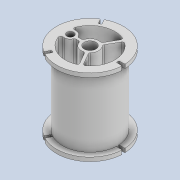
# Autodesk Inventor part: roller_3
Saved by Autodesk Inventor 2020 (Build 240168000, 168)
## iProperties
Created: 2021-09-21
Part Number: roller_3
Material: Generic
Document SubType Name: Modeling
Designer: Shuang Peng
Density: 1 g/cm^3
Appearance: Default
Author: Shuang Peng
Autodesk Inventor part; units mm, degrees
ref_plane "YZ Plane" through (0, 0, 0) normal (1, 0, 0) x (0, 1, 0)
ref_plane "XZ Plane" through (0, 0, 0) normal (0, 1, 0) x (-1, 0, 0)
ref_plane "XY Plane" through (0, 0, 0) normal (0, 0, 1) x (1, 0, 0)
sketch "Sketch1" plane through (0, 0, 0) normal (0, 1, 0) x (-1, 0, 0)
  circle A0 centre (0, 0) radius 7
  circle A1 centre (0, 0) radius 1.5
  circle A2 centre (0, 0) radius 2.2
  circle A3 centre (0, 0) radius 6.3
  line L0 (0, 0) -> (7, 0)
  line L1 (7, 0) -> (0, 0) construction
  line L2 (7, 0.35) -> (0, 0.35)
  line L3 (0, -0.35) -> (7, -0.35)
  arc A4 (7, -0.35) -> (7, 0.35) centre (7, 0) ccw
  arc A5 (0, 0.35) -> (0, -0.35) centre (0, 0) ccw
  line L4 (0.3031, 0.175) -> (-3.1969, 6.2372)
  line L5 (-3.8031, 5.8872) -> (-0.3031, -0.175)
  line L6 (-0.3031, 0.175) -> (-3.8031, -5.8872)
  line L7 (-3.1969, -6.2372) -> (0.3031, -0.175)
  line L8 (0, 0) -> (5, 0)
  circle A6 centre (5, 0) radius 1.5
  line L9 (5, 1.5) -> (6.1188, 1.5)
  line L10 (5, -1.5) -> (6.1188, -1.5)
  line L11 (5, 0) -> (5, -1.5)
  line L12 (5, 0) -> (5, 1.5)
  point P0 (3.5, 0)
  point P1 (-0.7829, 2.056)
  point P2 (-2.842, 5.6225)
  point P3 (3.5414, 0.35)
  point P4 (2.172, 0.35)
  point P5 (-1.3891, 1.706)
  point P6 (-1.3891, -1.706)
  point P7 (-3.4482, -5.2725)
  point P8 (-3.4482, 5.2725)
  point P9 (-2.842, -5.6225)
  point P10 (-0.7829, -2.056)
  point P11 (2.172, -0.35)
  point P12 (3.5414, -0.35)
  dimension "d0" = 14
  dimension "d1" = 3
  dimension "d2" = 0.7
  dimension "d3" = 0.7
  dimension "d4" = 3.5
  dimension "d5" = 0.7
  dimension "d8" = 360
  dimension "d10" = 5
  dimension "d11" = 3
  constraints: 28 end point, 8 point on circle, 6 centre point, 5 coincident, 4 tangent, 2 horizontal, 2 midpoint, 2 parallel, 1 collinear, 1 horizontal alignment, 1 perpendicular, 1 point on line, 1 vertical, 21 other
  measures "d1" diameter of A1
  measures "d2" radial gap between concentric circles of A1 A2
  measures "d4" distance of point (3.5, 0) L0.start
  measures "d5" diameter of A5
  measures "d10" distance of L0.start L8.end
  measures "d11" diameter of A6
extrude "Extrusion1" add sketch "Sketch1" along normal blind 19.5 contours L0 A6 L2 A0 | A0 L3 A6 L0 | L2 A6 A3 L4 A0 | A0 L7 A3 A6 L3 | A6 L3 A3 L0 | L0 A3 L2 A6 | L4 A3 L5 A0 | L2 A3 A6 | A0 L6 A3 L7 | A6 A3 L3 | L0 L12 L2 A3 | A3 L3 L11 L0 | L5 A3 L6 A0 | L4 A2 L5 A3 | L2 L12 A6 A3 | A6 L9 A3 | A3 L6 A2 L7 | A3 A6 L11 L3 | A3 L10 A6 | L11 L3 A6 L0 | L0 A6 L2 L12 | L4 A1 L5 A2 | A2 L2 A1 L4 | L2 A6 L12 | L7 A1 L3 A2 | A2 L6 A1 L7 | L11 A6 L3 | A6 L3 A2 L0 | L0 A2 L2 A6 | L5 A1 L6 A2 | A2 L0 A1 L2 | L3 A1 L0 A2
sketch "Sketch2" plane through (0, 19.5, 0) normal (0, 1, 0) x (1, 0, 0)
  circle A0 centre (0, 0) radius 7 projected
  line L0 (-3.5414, -0.35) -> (-2.172, -0.35) projected
  arc A1 (-2.172, -0.35) -> (0.7829, -2.056) centre (0, 0) ccw projected
  line L1 (0.7829, -2.056) -> (2.842, -5.6225) projected
  arc A2 (-6.1188, -1.5) -> (2.842, -5.6225) centre (0, 0) ccw projected
  line L2 (-6.1188, -1.5) -> (-5, -1.5) projected
  arc A3 (-5, -1.5) -> (-3.5414, -0.35) centre (-5, 0) ccw projected
  arc A4 (3.4482, -5.2725) -> (3.4482, 5.2725) centre (0, 0) ccw projected
  line L3 (3.4482, -5.2725) -> (1.3891, -1.706) projected
  arc A5 (1.3891, -1.706) -> (1.3891, 1.706) centre (0, 0) ccw projected
  line L4 (1.3891, 1.706) -> (3.4482, 5.2725) projected
  circle A6 centre (0, 0) radius 1.5 projected
  arc A7 (2.842, 5.6225) -> (-6.1188, 1.5) centre (0, 0) ccw projected
  line L5 (2.842, 5.6225) -> (0.7829, 2.056) projected
  arc A8 (0.7829, 2.056) -> (-2.172, 0.35) centre (0, 0) ccw projected
  line L6 (-2.172, 0.35) -> (-3.5414, 0.35) projected
  arc A9 (-3.5414, 0.35) -> (-5, 1.5) centre (-5, 0) ccw projected
  line L7 (-5, 1.5) -> (-6.1188, 1.5) projected
  circle A10 centre (-5, 0) radius 0.9
  dimension "d14" = 1.8
  constraints: 1 centre point, 1 coincident
  measures "d14" diameter of A10
extrude "Extrusion2" cut sketch "Sketch2" against normal blind 19.5 contours A10
sketch "Sketch3" plane through (0, 19.5, 0) normal (0, 1, 0) x (1, 0, 0)
  circle A0 centre (-5, 0) radius 0.9 projected
  circle A1 centre (0, 0) radius 7 projected
  line L0 (-3.5414, -0.35) -> (-2.172, -0.35) projected
  arc A2 (-2.172, -0.35) -> (0.7829, -2.056) centre (0, 0) ccw projected
  line L1 (0.7829, -2.056) -> (2.842, -5.6225) projected
  arc A3 (-6.1188, -1.5) -> (2.842, -5.6225) centre (0, 0) ccw projected
  line L2 (-6.1188, -1.5) -> (-5, -1.5) projected
  arc A4 (-5, -1.5) -> (-3.5414, -0.35) centre (-5, 0) ccw projected
  arc A5 (3.4482, -5.2725) -> (3.4482, 5.2725) centre (0, 0) ccw projected
  line L3 (3.4482, -5.2725) -> (1.3891, -1.706) projected
  arc A6 (1.3891, -1.706) -> (1.3891, 1.706) centre (0, 0) ccw projected
  line L4 (1.3891, 1.706) -> (3.4482, 5.2725) projected
  circle A7 centre (0, 0) radius 1.5 projected
  arc A8 (2.842, 5.6225) -> (-6.1188, 1.5) centre (0, 0) ccw projected
  line L5 (2.842, 5.6225) -> (0.7829, 2.056) projected
  arc A9 (0.7829, 2.056) -> (-2.172, 0.35) centre (0, 0) ccw projected
  line L6 (-2.172, 0.35) -> (-3.5414, 0.35) projected
  arc A10 (-3.5414, 0.35) -> (-5, 1.5) centre (-5, 0) ccw projected
  line L7 (-5, 1.5) -> (-6.1188, 1.5) projected
  circle A11 centre (0, 0) radius 8.5
  dimension "d17" = 1.5
  constraints: 1 centre point, 1 coincident
  measures "d17" radial gap between concentric circles of A1 A11
extrude "Extrusion3" add sketch "Sketch3" against normal blind 1 contours A11
sketch "Sketch4" plane through (0, 0, 0) normal (0, -1, 0) x (1, 0, 0)
  circle A0 centre (0, 0) radius 8.5 projected
  circle A1 centre (0, 0) radius 7 projected
extrude "Extrusion4" add sketch "Sketch4" against normal blind 1
sketch "Sketch5" plane through (0, 0, 0) normal (0, -1, 0) x (1, 0, 0)
  circle A0 centre (0, 0) radius 8.5 projected
  circle A1 centre (-5, 0) radius 0.9 projected
  line L0 (-3.5414, 0.35) -> (-2.172, 0.35) projected
  arc A2 (-3.5414, 0.35) -> (-5, 1.5) centre (-5, 0) ccw projected
  line L1 (-6.1188, 1.5) -> (-5, 1.5) projected
  arc A3 (2.842, 5.6225) -> (-6.1188, 1.5) centre (0, 0) ccw projected
  line L2 (0.7829, 2.056) -> (2.842, 5.6225) projected
  arc A4 (0.7829, 2.056) -> (-2.172, 0.35) centre (0, 0) ccw projected
  arc A5 (3.4482, -5.2725) -> (3.4482, 5.2725) centre (0, 0) ccw projected
  line L3 (1.3891, -1.706) -> (3.4482, -5.2725) projected
  arc A6 (1.3891, -1.706) -> (1.3891, 1.706) centre (0, 0) ccw projected
  line L4 (3.4482, 5.2725) -> (1.3891, 1.706) projected
  circle A7 centre (0, 0) radius 1.5 projected
  arc A8 (-6.1188, -1.5) -> (2.842, -5.6225) centre (0, 0) ccw projected
  line L5 (-5, -1.5) -> (-6.1188, -1.5) projected
  arc A9 (-5, -1.5) -> (-3.5414, -0.35) centre (-5, 0) ccw projected
  line L6 (-2.172, -0.35) -> (-3.5414, -0.35) projected
  arc A10 (-2.172, -0.35) -> (0.7829, -2.056) centre (0, 0) ccw projected
  line L7 (2.842, -5.6225) -> (0.7829, -2.056) projected
  line L8 (0, 0) -> (-3.15, 5.456)
  line L9 (-4.65, 8.054) -> (-1.65, 2.8579) construction
  line L10 (-4.9531, 7.879) -> (-1.9531, 2.6829)
  line L11 (-1.3469, 3.0329) -> (-4.3469, 8.229)
  arc A11 (-4.3469, 8.229) -> (-4.9531, 7.879) centre (-4.65, 8.054) ccw
  arc A12 (-1.9531, 2.6829) -> (-1.3469, 3.0329) centre (-1.65, 2.8579) ccw
  circle A13 centre (0, 0) radius 7 projected
  point P0 (-3.7987, 5.8796)
  point P1 (-3.1925, 6.2296)
  point P2 (-3.9433, 7.53)
  point P3 (-4.5495, 7.18)
  dimension "d22" = 60
  dimension "d23" = 3
  dimension "d24" = 0.7
  constraints: 10 end point, 5 point on circle, 4 tangent, 2 centre point, 1 midpoint, 1 parallel, 1 point on line
  measures "d22" angle of L0 L8
  measures "d23" distance of L8.end L9.end
  measures "d24" diameter of A12
extrude "Extrusion5" cut sketch "Sketch5" against normal blind 20 contours L11 A13 L10 A0 picked at (-3.5114, 6.6264)
pattern_circular "Circular Pattern1" count 3 over 360 about axis through (0, 0, 0) along (0, 1, 0) of "Extrusion5"
fillet "Fillet1" radius 0.2 24 edges at (-3.1925, 0.5, -6.2296) (-3.7987, 0.5, -5.8796) (-3.9433, 0.5, -7.53) (-4.5495, 0.5, -7.18) (-3.1925, 0.5, 6.2296) (-3.7987, 0.5, 5.8796) (-3.9433, 0.5, 7.53) (-4.5495, 0.5, 7.18) (6.9912, 0.5, -0.35) (6.9912, 0.5, 0.35) (8.4928, 0.5, -0.35) (8.4928, 0.5, 0.35) (-3.9433, 19, 7.53) (-4.5495, 19, 7.18) (-3.7987, 19, 5.8796) (-3.1925, 19, 6.2296) (8.4928, 19, 0.35) (8.4928, 19, -0.35) (6.9912, 19, 0.35) (6.9912, 19, -0.35) (-3.7987, 19, -5.8796) (-3.1925, 19, -6.2296) (-4.5495, 19, -7.18) (-3.9433, 19, -7.53)
fillet "Fillet2" radius 0.5 14 edges at (2.842, 9.75, -5.6225) (3.4482, 9.75, -5.2725) (2.842, 9.75, 5.6225) (3.4482, 9.75, 5.2725) (-6.1188, 9.75, 1.5) (-6.1188, 9.75, -1.5) (-3.5414, 9.75, 0.35) (-3.5414, 9.75, -0.35) (-2.172, 9.75, 0.35) (-2.172, 9.75, -0.35) (0.7829, 9.75, 2.056) (1.3891, 9.75, 1.706) (0.7829, 9.75, -2.056) (1.3891, 9.75, -1.706)
body "Solid1"
